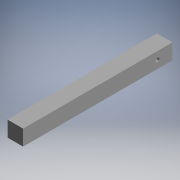
# Autodesk Inventor part: 30x30 pillars
Saved by Autodesk Inventor 2019 (Build 230136000, 136)
## iProperties
Part Number: 30x30 pillars
Material: Generic
Document SubType Name: Modeling
Designer: Delta
Appearance: Default
Author: Delta
Autodesk Inventor part; units mm, degrees
ref_plane "YZ Plane" through (0, 0, 0) normal (1, 0, 0) x (0, 1, 0)
ref_plane "XZ Plane" through (0, 0, 0) normal (0, 1, 0) x (-1, 0, 0)
ref_plane "XY Plane" through (0, 0, 0) normal (0, 0, 1) x (1, 0, 0)
sketch "Sketch1" plane through (0, 0, 0) normal (0, 0, 1) x (1, 0, 0)
  line L0 (0, 0) -> (12.5, 0)
  line L1 (12.5, 0) -> (12.5, 12.5)
  line L2 (12.5, 12.5) -> (0, 12.5)
  line L3 (0, 12.5) -> (0, 0)
  dimension "d0" = 12.5
  dimension "d1" = 12.5
  constraints: 8 end point, 2 parallel, 1 horizontal, 1 perpendicular
  measures "d0" distance between parallel lines of L1 L3
  measures "d1" distance between parallel lines of L0 L2
extrude "Extrusion1" add sketch "Sketch1" along normal blind 120
sketch "Sketch2" plane through (12.5, 0, 0) normal (1, 0, 0) x (0, 0, -1)
  line L0 (0, 0) -> (0, 12.5) projected
  line L1 (0, 12.5) -> (-120, 12.5) projected
  line L2 (0, 0) -> (-120, 0) projected
  circle A0 centre (-12, 6.25) radius 1.5
  dimension "d4" = 12
  dimension "d5" = 12.5
  dimension "d6" = 6.25
  dimension "d7" = 3
  constraints: 1 centre point, 1 coincident
  measures "d4" distance from line of L0 point (-12, 6.25)
  measures "d5" distance between parallel lines of L1 L2
  measures "d6" distance from line of L1 point (-12, 6.25)
  measures "d7" diameter of A0
extrude "Extrusion2" cut sketch "Sketch2" against normal through all
equation "\"d0\" = d1"
equation "\"d6\" = 0.5 * d5"
body "Solid1"
